big_button (Autodesk Fusion 360 design; units mm, degrees)
Autodesk Fusion 360 part; units mm, degrees
sketch "Sketch1" plane through (0, 0, 0) normal (1, 0, 0) x (0, 1, 0)
  line L0 (0, 0) -> (-11.9, 0)
  line L1 (-11.9, 0) -> (-11.9, 11.9)
  line L2 (-11.9, 11.9) -> (0, 11.9)
  line L3 (0, 11.9) -> (0, 0)
  dimension "d1" = 11.9
  dimension "d2" = 11.9
  constraint horizontal L0
  constraint vertical L1
  constraint horizontal L2
  constraint vertical L3
  constraint coincident L0.start L3.end
  measures "d1" distance of L1.end L2.end
  measures "d2" distance of L0.end L1.end
extrude "Extrude1" add sketch "Sketch1" along normal blind 3.8
sketch "Sketch2" plane through (3.8, 0, 0) normal (1, 0, 0) x (0, 1, 0)
  line L0 (0, 11.9) -> (-11.9, 11.9)
  line L1 (-11.9, 11.9) -> (-11.9, 0)
  line L2 (-11.9, 0) -> (0, 0)
  line L3 (0, 0) -> (0, 11.9)
  line L4 (-5.95, 11.9) -> (-5.95, 0)
  line L5 (0, 5.95) -> (-11.9, 5.95)
  circle A0 centre (-5.95, 5.95) radius 3.35
  dimension "d5" = 6.7
  constraint midpoint L0 L4.start
  constraint midpoint L2 L4.end
  constraint midpoint L3 L5.start
  constraint midpoint L1 L5.end
  constraint midpoint L4 A0.centre
  measures "d5" diameter of A0
extrude "Extrude2" add sketch "Sketch2" along normal blind 2.8 contours L4 L5 A0 | L4 L5 A0 | L4 L5 A0 | L4 L5 A0
sketch "Sketch3" plane through (0, 0, 0) normal (0, 0, -1) x (1, 0, 0)
  line L0 (0, 11.9) -> (0, 0)
  line L1 (0, 0) -> (3.8, 0)
  line L2 (3.8, 0) -> (3.8, 11.9)
  line L3 (3.8, 11.9) -> (0, 11.9)
  line L4 (0.2, 9.3) -> (1.8, 9.3)
  line L5 (1.8, 9.3) -> (1.8, 2.6)
  line L6 (1.8, 2.6) -> (0.2, 2.6)
  line L7 (0.2, 2.6) -> (0.2, 9.3)
  dimension "d8" = 2.6
  dimension "d10" = 2.6
  dimension "d11" = 0.2
  dimension "d12" = 2
  constraint horizontal L4
  constraint vertical L5
  constraint horizontal L6
  constraint vertical L7
  measures "d8" distance of L1 L6
  measures "d10" distance of L3 L4
  measures "d11" distance of L0 L7
  measures "d12" distance of L2 L5
extrude "Extrude3" add sketch "Sketch3" along normal blind 4.6 contours L4 L5 L6 L7
equation "d10 = d8"
